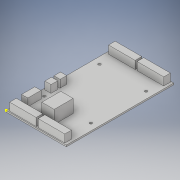
# Autodesk Inventor part: PCB
Saved by Autodesk Inventor 2018 (Build 220112000, 112)
## iProperties
Created: 2018-05-15
Part Number: PCB
Material: Generic
Document SubType Name: Modeling
Designer: alexs
Density: 1 g/cm^3
Appearance: Default
Author: alexs
Autodesk Inventor part; units mm, degrees
ref_plane "YZ Plane" through (0, 0, 0) normal (1, 0, 0) x (0, 1, 0)
ref_plane "XZ Plane" through (0, 0, 0) normal (0, 1, 0) x (-1, 0, 0)
ref_plane "XY Plane" through (0, 0, 0) normal (0, 0, 1) x (1, 0, 0)
sketch "Sketch1" plane through (0, 0, 0) normal (0, 0, 1) x (1, 0, 0)
  line L0 (0, 0) -> (63.23, 0)
  line L1 (63.23, 0) -> (63.23, 113)
  line L2 (63.23, 113) -> (0, 113)
  line L3 (0, 113) -> (0, 0)
  line L4 (7.115, 91) -> (56.115, 91) construction
  line L5 (56.115, 91) -> (56.115, 33) construction
  line L6 (56.115, 33) -> (7.115, 33) construction
  line L7 (7.115, 33) -> (7.115, 91) construction
  circle A0 centre (7.115, 91) radius 1.35
  circle A1 centre (56.115, 91) radius 1.35
  circle A2 centre (56.115, 33) radius 1.35
  circle A3 centre (7.115, 33) radius 1.35
  point P0 (31.615, 91)
  point P1 (31.615, 113)
  dimension "d0" = 63.23
  dimension "d1" = 113
  dimension "d2" = 49
  dimension "d3" = 58
  dimension "d4" = 2.7
  dimension "d5" = 22
  constraints: 16 end point, 4 centre point, 4 coincident, 4 parallel, 3 equal radius, 2 horizontal, 2 midpoint, 2 perpendicular, 1 vertical alignment
  measures "d0" distance of L2.end L1.end
  measures "d1" distance of L1.end L0.end
  measures "d2" distance of L5.end L6.end
  measures "d3" distance of L4.end L5.end
  measures "d4" diameter of A0
  measures "d5" distance between parallel lines of L4 L2
extrude "Extrusion1" add sketch "Sketch1" along normal blind 1.6
sketch "Sketch2" plane through (0, 0, 1.6) normal (0, 0, 1) x (1, 0, 0)
  point P0 (0, 0)
sketch "Sketch3" plane through (0, 0, 1.6) normal (0, 0, 1) x (1, 0, 0)
  line L0 (2.615, 112) -> (30.615, 112)
  line L1 (30.615, 112) -> (30.615, 105)
  line L2 (30.615, 105) -> (2.615, 105)
  line L3 (2.615, 105) -> (2.615, 112)
  line L4 (32.615, 112) -> (60.615, 112)
  line L5 (60.615, 112) -> (60.615, 105)
  line L6 (60.615, 105) -> (32.615, 105)
  line L7 (32.615, 105) -> (32.615, 112)
  line L8 (2.615, 1) -> (30.615, 1)
  line L9 (30.615, 1) -> (30.615, 8)
  line L10 (30.615, 8) -> (2.615, 8)
  line L11 (2.615, 8) -> (2.615, 1)
  line L12 (32.615, 1) -> (60.615, 1)
  line L13 (60.615, 1) -> (60.615, 8)
  line L14 (60.615, 8) -> (32.615, 8)
  line L15 (32.615, 8) -> (32.615, 1)
  line L16 (63.23, 113) -> (0, 113) construction
  line L17 (0, 0) -> (63.23, 0) construction
  line L18 (0, 113) -> (0, 0) construction
  dimension "d8" = 28
  dimension "d9" = 2
  dimension "d10" = 2
  dimension "d11" = 7
  dimension "d12" = 1
  dimension "d13" = 1
  dimension "d14" = 63.23
  dimension "d15" = 2.615
  dimension "d16" = 2.615
  constraints: 32 end point, 8 parallel, 4 equal length, 4 horizontal, 4 perpendicular, 3 collinear, 1 point on line
  measures "d8" distance of L0.start L0.end
  measures "d9" distance between parallel lines of L7 L1
  measures "d10" distance between parallel lines of L15 L9
  measures "d11" distance of L4.end L5.end
  measures "d12" distance between parallel lines of L17 L12
  measures "d13" distance between parallel lines of L16 L4
  measures "d14" distance of L16.start L16.end
  measures "d15" distance between parallel lines of L18 L3
  measures "d16" distance between parallel lines of L18 L11
extrude "Extrusion2" add sketch "Sketch3" along normal blind 8.3
sketch "Sketch4" plane through (0, 0, 1.6) normal (0, 0, 1) x (1, 0, 0)
  line L0 (1.6, 28.5) -> (8.1, 28.5)
  line L1 (8.1, 28.5) -> (8.1, 14.5)
  line L2 (8.1, 14.5) -> (1.6, 14.5)
  line L3 (1.6, 14.5) -> (1.6, 28.5)
  line L4 (0, 0) -> (63.23, 0) construction
  line L5 (0, 113) -> (0, 0) projected
  line L6 (1.6, 55.5) -> (8.1, 55.5)
  line L7 (8.1, 55.5) -> (8.1, 48.5)
  line L8 (8.1, 48.5) -> (1.6, 48.5)
  line L9 (1.6, 48.5) -> (1.6, 55.5)
  line L10 (1.6, 46) -> (8.1, 46)
  line L11 (8.1, 46) -> (8.1, 39)
  line L12 (8.1, 39) -> (1.6, 39)
  line L13 (1.6, 39) -> (1.6, 46)
  dimension "d19" = 6.5
  dimension "d20" = 14
  dimension "d21" = 28.5
  dimension "d22" = 1.6
  dimension "d30" = 7
  dimension "d31" = 7
  dimension "d32" = 10.5
  dimension "d33" = 2.5
  constraints: 24 end point, 7 parallel, 3 horizontal, 3 perpendicular, 2 point on line, 1 collinear
  measures "d19" distance of L0.start L0.end
  measures "d20" distance of L0.end L1.end
  measures "d21" distance between parallel lines of L4 L0
  measures "d22" distance between parallel lines of L5 L3
  measures "d30" distance of L6.end L7.end
  measures "d31" distance of L10.end L11.end
  measures "d32" distance between parallel lines of L0 L12
  measures "d33" distance between parallel lines of L10 L8
extrude "Extrusion3" add sketch "Sketch4" along normal blind 8
sketch "Sketch5" plane through (0, 0, 1.6) normal (0, 0, 1) x (1, 0, 0)
  line L0 (25.115, 32.3) -> (38.115, 32.3)
  line L1 (38.115, 32.3) -> (38.115, 12.3)
  line L2 (38.115, 12.3) -> (25.115, 12.3)
  line L3 (25.115, 12.3) -> (25.115, 32.3)
  line L4 (0, 0) -> (63.23, 0) construction
  point P0 (31.615, 12.3)
  point P1 (31.615, 0)
  dimension "d25" = 12.3
  dimension "d26" = 13
  dimension "d27" = 20
  constraints: 8 end point, 2 midpoint, 2 parallel, 1 horizontal, 1 perpendicular, 1 vertical alignment
  measures "d25" distance between parallel lines of L4 L2
  measures "d26" distance of L0.start L0.end
  measures "d27" distance of L0.end L1.end
extrude "Extrusion4" add sketch "Sketch5" along normal blind 13.8
equation "\"d10\" = d9"
equation "\"d13\" = d12"
equation "\"d15\" = -0.5 * d9 + 0.5 * d14 - d8"
equation "\"d16\" = d15"
equation "\"d31\" = d30"
body "Solid1"
